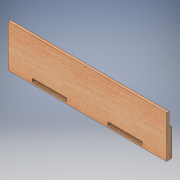
# Autodesk Inventor part: SkinnySideW
Saved by Autodesk Inventor 2016 (Build 200138000, 138)
## iProperties
Created: 2016-02-11
Part Number: SkinnySideW
Material: Wood (Birch)
Document SubType Name: Modeling
Designer: ron
Density: 0.55 g/cm^3
Appearance: Birch - Natural Polished
Mass: 828.134 g
Surface Area: 2264.58 cm^2
Volume: 1505.7 cm^3
Author: ron
Autodesk Inventor part; units mm, degrees
ref_plane "YZ Plane" through (0, 0, 0) normal (1, 0, 0) x (0, 1, 0)
ref_plane "XZ Plane" through (0, 0, 0) normal (0, 1, 0) x (-1, 0, 0)
ref_plane "XY Plane" through (0, 0, 0) normal (0, 0, 1) x (1, 0, 0)
sketch "Sketch1" plane through (0, 0, 0) normal (1, 0, 0) x (0, 1, 0)
  line L0 (0, 0) -> (155.1, 0)
  line L1 (155.1, 0) -> (155.1, -10)
  line L2 (0, -20) -> (0, 0)
  line L3 (155.1, -10) -> (101.6, -10)
  line L4 (101.6, -10) -> (101.6, -20)
  line L5 (101.6, -20) -> (0, -20)
  dimension "d0" = 53.5
  dimension "d1" = 155.1
  dimension "d2" = 10
  dimension "d3" = 10
  dimension "d4" = 20
  constraints: 12 end point, 3 horizontal, 2 parallel, 1 perpendicular
  measures "d0" distance of L1.end L3.end
  measures "d1" distance between parallel lines of L1 L2
  measures "d2" distance between parallel lines of L3 L5
  measures "d3" distance between parallel lines of L0 L3
  measures "d4" vertical distance of L4.end L0.end
extrude "Extrusion1" add sketch "Sketch1" along normal blind 584.6
ref_plane "Work Plane2" through (609.4222, 0, -20) normal (0, 0, -1) x (-1, 0, 0)
sketch "Sketch2" plane through (609.4222, 0, -20) normal (0, 0, -1) x (-1, 0, 0)
  line L0 (609.4222, 0) -> (609.4222, 155.1) projected
  line L1 (609.4222, 0) -> (609.4222, 6.35)
  line L2 (520.5222, 6.35) -> (520.5222, 19.05)
  line L3 (520.5222, 19.05) -> (393.1222, 19.05)
  line L4 (393.1222, 19.05) -> (393.1222, 6.35)
  line L5 (393.1222, 6.35) -> (240.7222, 6.35)
  line L6 (240.7222, 6.35) -> (240.7222, 19.05)
  line L7 (240.7222, 19.05) -> (113.7222, 19.05)
  line L8 (113.7222, 19.05) -> (113.7222, 6.35)
  line L9 (113.7222, 6.35) -> (240.7222, 6.35)
  line L10 (393.1222, 6.35) -> (520.5222, 6.35)
  line L11 (24.8222, 0) -> (24.8222, 101.6) projected
  dimension "d39" = 6.35
  dimension "d41" = 12.7
  dimension "d42" = 90
  dimension "d43" = 152.4
  dimension "d44" = 127
  dimension "d45" = 12.7
  dimension "d58" = 88.9
  constraints: 20 end point, 6 perpendicular, 2 point on line, 1 horizontal
  measures "d39" distance of L0.start L1.end
  measures "d41" distance of L2.start L2.end
  measures "d42" angle of L3 L2
  measures "d43" distance of L4.end L5.end
  measures "d44" distance of L6.end L7.end
  measures "d45" distance of L5.end L6.end
  measures "d58" distance between parallel lines of L11 L8
ref_plane "Work Plane1" through (609.4222, 0, -20) normal (0, 0, -1) x (-1, 0, 0)
sketch "Sketch3" plane through (609.4222, 0, -20) normal (0, 0, -1) x (-1, 0, 0)
  line L0 (609.4222, 0) -> (609.4222, 155.1)
  line L1 (609.4222, 0) -> (609.4222, 6.35)
  line L2 (520.5222, 6.35) -> (520.5222, 19.05)
  line L3 (520.5222, 19.05) -> (393.1222, 19.05)
  line L4 (393.1222, 19.05) -> (393.1222, 6.35)
  line L5 (393.1222, 6.35) -> (240.7222, 6.35)
  line L6 (240.7222, 6.35) -> (240.7222, 19.05)
  line L7 (240.7222, 19.05) -> (113.7222, 19.05)
  line L8 (113.7222, 19.05) -> (113.7222, 6.35)
  line L9 (113.7222, 6.35) -> (240.7222, 6.35)
  line L10 (393.1222, 6.35) -> (520.5222, 6.35)
  line L11 (24.8222, 0) -> (24.8222, 101.6) projected
  dimension "d46" = 6.35
  dimension "d48" = 12.7
  dimension "d49" = 90
  dimension "d50" = 152.4
  dimension "d51" = 127
  dimension "d52" = 12.7
  dimension "d57" = 88.9
  constraints: 22 end point, 6 perpendicular, 2 point on line, 1 horizontal
  measures "d46" distance of L0.start L1.end
  measures "d48" distance of L2.start L2.end
  measures "d49" angle of L3 L2
  measures "d50" distance of L4.end L5.end
  measures "d51" distance of L6.end L7.end
  measures "d52" distance of L5.end L6.end
  measures "d57" distance between parallel lines of L11 L8
extrude "Extrusion4" cut sketch "Sketch3" against normal blind 127 contours L9 L8 L7 L6
extrude "Extrusion5" cut sketch "Sketch2" against normal blind 127 contours L10 L4 L3 L2
body "Solid1"
